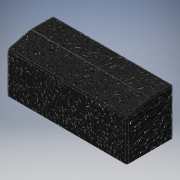
# Autodesk Inventor part: SPUST
Saved by Autodesk Inventor 2017 SP1 (Build 210196100, 196)
## iProperties
Created: 2021-03-15
Part Number: SPUST
Material: Tworzywo sztuczne, nieprzezroczyste czarne
Document SubType Name: Modeling
Designer: Administrator
Density: 0.952 g/cm^3
Appearance: Chropowaty, teksturowany - czarny
Author: Administrator
Autodesk Inventor part; units mm, degrees
ref_plane "YZ Plane" through (0, 0, 0) normal (1, 0, 0) x (0, 1, 0)
ref_plane "XZ Plane" through (0, 0, 0) normal (0, 1, 0) x (-1, 0, 0)
ref_plane "XY Plane" through (0, 0, 0) normal (0, 0, 1) x (1, 0, 0)
sketch "Szkic1" plane through (0, 0, 0) normal (0, 0, 1) x (1, 0, 0)
  line L0 (10.35, -71.2) -> (-10.35, -71.2)
  line L1 (-10.35, -71.2) -> (-10.35, -63.2)
  line L2 (-10.35, -63.2) -> (10.35, -63.2)
  line L3 (10.35, -63.2) -> (10.35, -71.2)
  constraints: 8 end point, 2 parallel, 1 horizontal, 1 perpendicular
extrude "Wyciągnięcie proste1" add sketch "Szkic1" along normal blind 5 and the other way blind 3
sketch "Szkic2" plane through (-10.35, -71.2, 5) normal (-1, 0, 0) x (0, 0, 1)
  line L0 (0, 0) -> (0, 4)
  line L1 (0, 4) -> (-1, 0)
  line L2 (0, 0) -> (-1, 0)
  point P0 (-5, 71.2)
  constraints: 6 end point
extrude "Wyciągnięcie proste2" cut sketch "Szkic2" against normal up to next
fillet "Zaokrąglenie1" radius 0.25 11 edges at (-10.35, -65.2, 5) (-10.35, -69.2, 4.5) (10.35, -69.2, 4.5) (10.35, -65.2, 5) (0, -67.2, 5) (0, -71.2, 4) (-10.35, -71.2, 0.5) (10.35, -71.2, 0.5) (-10.35, -63.2, 1) (0, -63.2, 5) (10.35, -63.2, 1)
